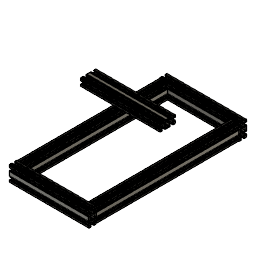
Frame (Autodesk Fusion 360 design; units mm, degrees)
part number: 2026-06-05-11-46-41-486
Autodesk Fusion 360 part; units mm, degrees
(part 1 of 2)
ref_plane "WorkPlane1" through (0, 20, 0) normal (0, 1, 0) x (0, 0, 1)
sketch "Sketch4" plane through (0, 20, 0) normal (0, 1, 0) x (1, 0, 0)
  line L0 (5.5, -26.5607) -> (5.5, -29.7925)
  line L1 (18.5, -27) -> (18.5, -24.05)
  line L2 (6.5607, -34.5) -> (9.7925, -34.5)
  line L3 (0, -26.5) -> (0, -13.5)
  line L4 (0.5, -27) -> (0.5, -26.5)
  line L5 (15.95, -17.0107) -> (15.95, -22.9893)
  line L6 (0, -33.5) -> (0.5, -33.5)
  line L7 (13.4393, -34.5) -> (10.2075, -34.5)
  line L8 (20, -33.5) -> (19.5, -33.5)
  line L9 (13.5, -40) -> (13.5, -39.5)
  line L10 (18.5, -35.95) -> (17.0107, -35.95)
  line L11 (2.9893, -35.95) -> (5.5, -33.4393)
  line L12 (0, -38.5) -> (0, -33.5)
  line L13 (19.5, -33) -> (18.5, -33)
  line L14 (4.05, -38.5) -> (4.05, -37.0107)
  line L15 (15.95, -22.9893) -> (13.4393, -25.5)
  line L16 (4.05, -17.0107) -> (4.05, -22.9893)
  line L17 (1.5, -24.05) -> (2.9893, -24.05)
  line L18 (15.95, -38.5) -> (15.95, -37.0107)
  line L19 (7, -38.5) -> (4.05, -38.5)
  line L20 (19.5, -26.5) -> (19.5, -27)
  line L21 (19.5, -33) -> (19.5, -33.5)
  line L22 (18.5, -33) -> (18.5, -35.95)
  line L23 (13, -39.5) -> (13, -38.5)
  line L24 (6.5, -40) -> (1.5, -40)
  line L25 (20, -33.5) -> (20, -38.5)
  line L26 (14.5, -33.4393) -> (14.5, -30.2075)
  line L27 (15.95, -37.0107) -> (13.4393, -34.5)
  line L28 (18.5, -24.05) -> (17.0107, -24.05)
  line L29 (5.5, -33.4393) -> (5.5, -30.2075)
  line L30 (7, -39.5) -> (6.5, -39.5)
  line L31 (4.05, -22.9893) -> (6.5607, -25.5)
  line L32 (17.0107, -35.95) -> (14.5, -33.4393)
  line L33 (0, -26.5) -> (0.5, -26.5)
  line L34 (1.5, -33) -> (1.5, -35.95)
  line L35 (1.5, -35.95) -> (2.9893, -35.95)
  line L36 (13, -38.5) -> (15.95, -38.5)
  line L37 (0.5, -33.5) -> (0.5, -33)
  line L38 (6.5607, -25.5) -> (9.7925, -25.5)
  line L39 (13.5, -39.5) -> (13, -39.5)
  line L40 (2.9893, -24.05) -> (5.5, -26.5607)
  line L41 (20, -26.5) -> (19.5, -26.5)
  line L42 (7, -39.5) -> (7, -38.5)
  line L43 (6.5, -40) -> (6.5, -39.5)
  line L44 (1.5, -27) -> (1.5, -24.05)
  line L45 (4.05, -37.0107) -> (6.5607, -34.5)
  line L46 (19.5, -27) -> (18.5, -27)
  line L47 (0.5, -33) -> (1.5, -33)
  line L48 (20, -13.5) -> (20, -26.5)
  line L49 (17.0107, -24.05) -> (14.5, -26.5607)
  line L50 (0.5, -27) -> (1.5, -27)
  line L51 (18.5, -40) -> (13.5, -40)
  line L52 (13.4393, -25.5) -> (10.2075, -25.5)
  line L53 (14.5, -26.5607) -> (14.5, -29.7925)
  line L54 (6.5, 0) -> (6.5, -0.5)
  line L55 (13, -0.5) -> (13.5, -0.5)
  line L56 (0.5, -7) -> (0.5, -6.5)
  line L57 (6.5607, -14.5) -> (9.7925, -14.5)
  line L58 (5.5, -13.4393) -> (5.5, -10.2075)
  line L59 (14.5, -13.4393) -> (14.5, -10.2075)
  line L60 (13.4393, -5.5) -> (10.2075, -5.5)
  line L61 (20, -1.5) -> (20, -6.5)
  line L62 (0, -6.5) -> (0.5, -6.5)
  line L63 (15.95, -17.0107) -> (13.4393, -14.5)
  line L64 (1.5, -7) -> (1.5, -4.05)
  line L65 (13.5, 0) -> (13.5, -0.5)
  line L66 (6.5607, -5.5) -> (9.7925, -5.5)
  line L67 (18.5, -4.05) -> (17.0107, -4.05)
  line L68 (7, -0.5) -> (7, -1.5)
  line L69 (4.05, -2.9893) -> (6.5607, -5.5)
  line L70 (6.5, -0.5) -> (7, -0.5)
  line L71 (19.5, -6.5) -> (19.5, -7)
  line L72 (13, -1.5) -> (15.95, -1.5)
  line L73 (0.5, -7) -> (1.5, -7)
  line L74 (19.5, -7) -> (18.5, -7)
  line L75 (13.5, 0) -> (18.5, 0)
  line L76 (14.5, -6.5607) -> (14.5, -9.7925)
  line L77 (18.5, -13) -> (18.5, -15.95)
  line L78 (19.5, -13) -> (18.5, -13)
  line L79 (1.5, 0) -> (6.5, 0)
  line L80 (18.5, -15.95) -> (17.0107, -15.95)
  line L81 (1.5, -15.95) -> (2.9893, -15.95)
  line L82 (19.5, -13) -> (19.5, -13.5)
  line L83 (15.95, -2.9893) -> (13.4393, -5.5)
  line L84 (0.5, -13) -> (1.5, -13)
  line L85 (1.5, -4.05) -> (2.9893, -4.05)
  line L86 (18.5, -7) -> (18.5, -4.05)
  line L87 (1.5, -13) -> (1.5, -15.95)
  line L88 (4.05, -17.0107) -> (6.5607, -14.5)
  line L89 (2.9893, -15.95) -> (5.5, -13.4393)
  line L90 (13.4393, -14.5) -> (10.2075, -14.5)
  line L91 (7, -1.5) -> (4.05, -1.5)
  line L92 (13, -0.5) -> (13, -1.5)
  line L93 (17.0107, -4.05) -> (14.5, -6.5607)
  line L94 (15.95, -1.5) -> (15.95, -2.9893)
  line L95 (20, -6.5) -> (19.5, -6.5)
  line L96 (17.0107, -15.95) -> (14.5, -13.4393)
  line L97 (0.5, -13.5) -> (0.5, -13)
  line L98 (20, -13.5) -> (19.5, -13.5)
  line L99 (2.9893, -4.05) -> (5.5, -6.5607)
  line L100 (0, -6.5) -> (0, -1.5)
  line L101 (0, -13.5) -> (0.5, -13.5)
  line L102 (5.5, -6.5607) -> (5.5, -9.7925)
  line L103 (4.05, -1.5) -> (4.05, -2.9893)
  circle A0 centre (10, -30) radius 2.74
  circle A1 centre (10, -10) radius 2.74
  arc A2 (9.7925, -25.5) -> (10.2075, -25.5) centre (10, -25.5) ccw
  arc A3 (18.5, -40) -> (20, -38.5) centre (18.5, -38.5) ccw
  arc A4 (14.5, -29.7925) -> (14.5, -30.2075) centre (14.5, -30) ccw
  arc A5 (0, -38.5) -> (1.5, -40) centre (1.5, -38.5) ccw
  arc A6 (5.5, -30.2075) -> (5.5, -29.7925) centre (5.5, -30) ccw
  arc A7 (10.2075, -34.5) -> (9.7925, -34.5) centre (10, -34.5) ccw
  arc A8 (9.7925, -5.5) -> (10.2075, -5.5) centre (10, -5.5) ccw
  arc A9 (20, -1.5) -> (18.5, 0) centre (18.5, -1.5) ccw
  arc A10 (10.2075, -14.5) -> (9.7925, -14.5) centre (10, -14.5) ccw
  arc A11 (5.5, -10.2075) -> (5.5, -9.7925) centre (5.5, -10) ccw
  arc A12 (14.5, -9.7925) -> (14.5, -10.2075) centre (14.5, -10) ccw
  arc A13 (1.5, 0) -> (0, -1.5) centre (1.5, -1.5) ccw
  line L104 (184.05, -17.0107) -> (184.05, -22.9893)
  line L105 (200, -13.5) -> (200, -26.5)
  line L106 (180, -26.5) -> (180, -13.5)
  line L107 (180.5, -7) -> (180.5, -6.5)
  line L108 (186.5, -40) -> (186.5, -39.5)
  line L109 (200, -26.5) -> (199.5, -26.5)
  line L110 (180.5, -33) -> (181.5, -33)
  line L111 (180, -6.5) -> (180, -1.5)
  line L112 (193.4393, -34.5) -> (190.2075, -34.5)
  line L113 (185.5, -13.4393) -> (185.5, -10.2075)
  line L114 (193, -1.5) -> (195.95, -1.5)
  line L115 (182.9893, -35.95) -> (185.5, -33.4393)
  arc A14 (190.2075, -34.5) -> (189.7925, -34.5) centre (190, -34.5) ccw
  line L116 (181.5, -35.95) -> (182.9893, -35.95)
  line L117 (180, -13.5) -> (180.5, -13.5)
  line L118 (181.5, -15.95) -> (182.9893, -15.95)
  line L119 (186.5, -0.5) -> (187, -0.5)
  line L120 (193.5, -39.5) -> (193, -39.5)
  arc A15 (194.5, -9.7925) -> (194.5, -10.2075) centre (194.5, -10) ccw
  line L121 (199.5, -33) -> (199.5, -33.5)
  line L122 (198.5, -13) -> (198.5, -15.95)
  line L123 (195.95, -17.0107) -> (193.4393, -14.5)
  line L124 (197.0107, -24.05) -> (194.5, -26.5607)
  line L125 (180.5, -13) -> (181.5, -13)
  line L126 (199.5, -7) -> (198.5, -7)
  line L127 (181.5, 0) -> (186.5, 0)
  line L128 (180.5, -27) -> (181.5, -27)
  line L129 (181.5, -27) -> (181.5, -24.05)
  line L130 (185.5, -26.5607) -> (185.5, -29.7925)
  line L131 (197.0107, -15.95) -> (194.5, -13.4393)
  line L132 (199.5, -26.5) -> (199.5, -27)
  line L133 (181.5, -7) -> (181.5, -4.05)
  circle A16 centre (190, -10) radius 2.74
  arc A17 (200, -1.5) -> (198.5, 0) centre (198.5, -1.5) ccw
  arc A18 (198.5, -40) -> (200, -38.5) centre (198.5, -38.5) ccw
  line L134 (195.95, -1.5) -> (195.95, -2.9893)
  line L135 (182.9893, -15.95) -> (185.5, -13.4393)
  line L136 (200, -33.5) -> (200, -38.5)
  line L137 (184.05, -2.9893) -> (186.5607, -5.5)
  line L138 (193.5, -40) -> (193.5, -39.5)
  line L139 (182.9893, -24.05) -> (185.5, -26.5607)
  line L140 (187, -0.5) -> (187, -1.5)
  line L141 (180.5, -13.5) -> (180.5, -13)
  line L142 (186.5, 0) -> (186.5, -0.5)
  arc A19 (185.5, -30.2075) -> (185.5, -29.7925) centre (185.5, -30) ccw
  line L143 (197.0107, -35.95) -> (194.5, -33.4393)
  line L144 (198.5, -24.05) -> (197.0107, -24.05)
  arc A20 (189.7925, -5.5) -> (190.2075, -5.5) centre (190, -5.5) ccw
  line L145 (198.5, -15.95) -> (197.0107, -15.95)
  line L146 (186.5607, -5.5) -> (189.7925, -5.5)
  line L147 (198.5, -7) -> (198.5, -4.05)
  line L148 (198.5, -4.05) -> (197.0107, -4.05)
  line L149 (193, -39.5) -> (193, -38.5)
  arc A21 (185.5, -10.2075) -> (185.5, -9.7925) centre (185.5, -10) ccw
  line L150 (194.5, -13.4393) -> (194.5, -10.2075)
  line L151 (180, -38.5) -> (180, -33.5)
  line L152 (199.5, -33) -> (198.5, -33)
  line L153 (199.5, -13) -> (199.5, -13.5)
  line L154 (184.05, -37.0107) -> (186.5607, -34.5)
  line L155 (180, -26.5) -> (180.5, -26.5)
  line L156 (180, -33.5) -> (180.5, -33.5)
  line L157 (198.5, -35.95) -> (197.0107, -35.95)
  line L158 (193.4393, -5.5) -> (190.2075, -5.5)
  line L159 (180.5, -33.5) -> (180.5, -33)
  line L160 (198.5, -27) -> (198.5, -24.05)
  line L161 (186.5607, -25.5) -> (189.7925, -25.5)
  line L162 (181.5, -4.05) -> (182.9893, -4.05)
  line L163 (199.5, -27) -> (198.5, -27)
  line L164 (180, -6.5) -> (180.5, -6.5)
  line L165 (184.05, -17.0107) -> (186.5607, -14.5)
  line L166 (193, -0.5) -> (193.5, -0.5)
  line L167 (186.5, -40) -> (181.5, -40)
  line L168 (187, -1.5) -> (184.05, -1.5)
  line L169 (194.5, -26.5607) -> (194.5, -29.7925)
  line L170 (199.5, -13) -> (198.5, -13)
  line L171 (181.5, -24.05) -> (182.9893, -24.05)
  line L172 (193.5, 0) -> (198.5, 0)
  line L173 (182.9893, -4.05) -> (185.5, -6.5607)
  line L174 (195.95, -22.9893) -> (193.4393, -25.5)
  line L175 (180.5, -27) -> (180.5, -26.5)
  line L176 (181.5, -13) -> (181.5, -15.95)
  arc A22 (180, -38.5) -> (181.5, -40) centre (181.5, -38.5) ccw
  line L177 (195.95, -2.9893) -> (193.4393, -5.5)
  line L178 (195.95, -38.5) -> (195.95, -37.0107)
  arc A23 (194.5, -29.7925) -> (194.5, -30.2075) centre (194.5, -30) ccw
  line L179 (194.5, -6.5607) -> (194.5, -9.7925)
  line L180 (197.0107, -4.05) -> (194.5, -6.5607)
  line L181 (193.4393, -25.5) -> (190.2075, -25.5)
  line L182 (181.5, -33) -> (181.5, -35.95)
  line L183 (187, -39.5) -> (187, -38.5)
  line L184 (184.05, -22.9893) -> (186.5607, -25.5)
  line L185 (193.4393, -14.5) -> (190.2075, -14.5)
  line L186 (184.05, -1.5) -> (184.05, -2.9893)
  line L187 (200, -13.5) -> (199.5, -13.5)
  line L188 (187, -38.5) -> (184.05, -38.5)
  line L189 (184.05, -38.5) -> (184.05, -37.0107)
  arc A24 (189.7925, -25.5) -> (190.2075, -25.5) centre (190, -25.5) ccw
  line L190 (195.95, -17.0107) -> (195.95, -22.9893)
  line L191 (198.5, -40) -> (193.5, -40)
  line L192 (186.5607, -14.5) -> (189.7925, -14.5)
  line L193 (194.5, -33.4393) -> (194.5, -30.2075)
  circle A25 centre (190, -30) radius 2.74
  line L194 (185.5, -33.4393) -> (185.5, -30.2075)
  line L195 (193, -0.5) -> (193, -1.5)
  line L196 (185.5, -6.5607) -> (185.5, -9.7925)
  arc A26 (181.5, 0) -> (180, -1.5) centre (181.5, -1.5) ccw
  line L197 (198.5, -33) -> (198.5, -35.95)
  line L198 (193, -38.5) -> (195.95, -38.5)
  line L199 (199.5, -6.5) -> (199.5, -7)
  line L200 (187, -39.5) -> (186.5, -39.5)
  line L201 (180.5, -7) -> (181.5, -7)
  line L202 (193.5, 0) -> (193.5, -0.5)
  arc A27 (190.2075, -14.5) -> (189.7925, -14.5) centre (190, -14.5) ccw
  line L203 (195.95, -37.0107) -> (193.4393, -34.5)
  line L204 (200, -33.5) -> (199.5, -33.5)
  line L205 (200, -1.5) -> (200, -6.5)
  line L206 (186.5607, -34.5) -> (189.7925, -34.5)
  line L207 (200, -6.5) -> (199.5, -6.5)
sketch "Sketch5" plane through (0, 0, 0) normal (1, 0, 0) x (0, 1, 0)
  line L0 (5.5, 13.4393) -> (5.5, 10.2075)
  line L1 (18.5, 13) -> (18.5, 15.95)
  line L2 (6.5607, 5.5) -> (9.7925, 5.5)
  line L3 (0, 13.5) -> (0, 26.5)
  line L4 (0.5, 13) -> (0.5, 13.5)
  line L5 (15.95, 22.9893) -> (15.95, 17.0107)
  line L6 (0, 6.5) -> (0.5, 6.5)
  line L7 (13.4393, 5.5) -> (10.2075, 5.5)
  line L8 (20, 6.5) -> (19.5, 6.5)
  line L9 (13.5, 0) -> (13.5, 0.5)
  line L10 (18.5, 4.05) -> (17.0107, 4.05)
  line L11 (2.9893, 4.05) -> (5.5, 6.5607)
  line L12 (0, 1.5) -> (0, 6.5)
  line L13 (19.5, 7) -> (18.5, 7)
  line L14 (4.05, 1.5) -> (4.05, 2.9893)
  line L15 (15.95, 17.0107) -> (13.4393, 14.5)
  line L16 (4.05, 22.9893) -> (4.05, 17.0107)
  line L17 (1.5, 15.95) -> (2.9893, 15.95)
  line L18 (15.95, 1.5) -> (15.95, 2.9893)
  line L19 (7, 1.5) -> (4.05, 1.5)
  line L20 (19.5, 13.5) -> (19.5, 13)
  line L21 (19.5, 7) -> (19.5, 6.5)
  line L22 (18.5, 7) -> (18.5, 4.05)
  line L23 (13, 0.5) -> (13, 1.5)
  line L24 (6.5, 0) -> (1.5, 0)
  line L25 (20, 6.5) -> (20, 1.5)
  line L26 (14.5, 6.5607) -> (14.5, 9.7925)
  line L27 (15.95, 2.9893) -> (13.4393, 5.5)
  line L28 (18.5, 15.95) -> (17.0107, 15.95)
  line L29 (5.5, 6.5607) -> (5.5, 9.7925)
  line L30 (7, 0.5) -> (6.5, 0.5)
  line L31 (4.05, 17.0107) -> (6.5607, 14.5)
  line L32 (17.0107, 4.05) -> (14.5, 6.5607)
  line L33 (0, 13.5) -> (0.5, 13.5)
  line L34 (1.5, 7) -> (1.5, 4.05)
  line L35 (1.5, 4.05) -> (2.9893, 4.05)
  line L36 (13, 1.5) -> (15.95, 1.5)
  line L37 (0.5, 6.5) -> (0.5, 7)
  line L38 (6.5607, 14.5) -> (9.7925, 14.5)
  line L39 (13.5, 0.5) -> (13, 0.5)
  line L40 (2.9893, 15.95) -> (5.5, 13.4393)
  line L41 (20, 13.5) -> (19.5, 13.5)
  line L42 (7, 0.5) -> (7, 1.5)
  line L43 (6.5, 0) -> (6.5, 0.5)
  line L44 (1.5, 13) -> (1.5, 15.95)
  line L45 (4.05, 2.9893) -> (6.5607, 5.5)
  line L46 (19.5, 13) -> (18.5, 13)
  line L47 (0.5, 7) -> (1.5, 7)
  line L48 (20, 26.5) -> (20, 13.5)
  line L49 (17.0107, 15.95) -> (14.5, 13.4393)
  line L50 (0.5, 13) -> (1.5, 13)
  line L51 (18.5, 0) -> (13.5, 0)
  line L52 (13.4393, 14.5) -> (10.2075, 14.5)
  line L53 (14.5, 13.4393) -> (14.5, 10.2075)
  line L54 (6.5, 40) -> (6.5, 39.5)
  line L55 (13, 39.5) -> (13.5, 39.5)
  line L56 (0.5, 33) -> (0.5, 33.5)
  line L57 (6.5607, 25.5) -> (9.7925, 25.5)
  line L58 (5.5, 26.5607) -> (5.5, 29.7925)
  line L59 (14.5, 26.5607) -> (14.5, 29.7925)
  line L60 (13.4393, 34.5) -> (10.2075, 34.5)
  line L61 (20, 38.5) -> (20, 33.5)
  line L62 (0, 33.5) -> (0.5, 33.5)
  line L63 (15.95, 22.9893) -> (13.4393, 25.5)
  line L64 (1.5, 33) -> (1.5, 35.95)
  line L65 (13.5, 40) -> (13.5, 39.5)
  line L66 (6.5607, 34.5) -> (9.7925, 34.5)
  line L67 (18.5, 35.95) -> (17.0107, 35.95)
  line L68 (7, 39.5) -> (7, 38.5)
  line L69 (4.05, 37.0107) -> (6.5607, 34.5)
  line L70 (6.5, 39.5) -> (7, 39.5)
  line L71 (19.5, 33.5) -> (19.5, 33)
  line L72 (13, 38.5) -> (15.95, 38.5)
  line L73 (0.5, 33) -> (1.5, 33)
  line L74 (19.5, 33) -> (18.5, 33)
  line L75 (13.5, 40) -> (18.5, 40)
  line L76 (14.5, 33.4393) -> (14.5, 30.2075)
  line L77 (18.5, 27) -> (18.5, 24.05)
  line L78 (19.5, 27) -> (18.5, 27)
  line L79 (1.5, 40) -> (6.5, 40)
  line L80 (18.5, 24.05) -> (17.0107, 24.05)
  line L81 (1.5, 24.05) -> (2.9893, 24.05)
  line L82 (19.5, 27) -> (19.5, 26.5)
  line L83 (15.95, 37.0107) -> (13.4393, 34.5)
  line L84 (0.5, 27) -> (1.5, 27)
  line L85 (1.5, 35.95) -> (2.9893, 35.95)
  line L86 (18.5, 33) -> (18.5, 35.95)
  line L87 (1.5, 27) -> (1.5, 24.05)
  line L88 (4.05, 22.9893) -> (6.5607, 25.5)
  line L89 (2.9893, 24.05) -> (5.5, 26.5607)
  line L90 (13.4393, 25.5) -> (10.2075, 25.5)
  line L91 (7, 38.5) -> (4.05, 38.5)
  line L92 (13, 39.5) -> (13, 38.5)
  line L93 (17.0107, 35.95) -> (14.5, 33.4393)
  line L94 (15.95, 38.5) -> (15.95, 37.0107)
  line L95 (20, 33.5) -> (19.5, 33.5)
  line L96 (17.0107, 24.05) -> (14.5, 26.5607)
  line L97 (0.5, 26.5) -> (0.5, 27)
  line L98 (20, 26.5) -> (19.5, 26.5)
  line L99 (2.9893, 35.95) -> (5.5, 33.4393)
  line L100 (0, 33.5) -> (0, 38.5)
  line L101 (0, 26.5) -> (0.5, 26.5)
  line L102 (5.5, 33.4393) -> (5.5, 30.2075)
  line L103 (4.05, 38.5) -> (4.05, 37.0107)
  circle A0 centre (10, 10) radius 2.74
  circle A1 centre (10, 30) radius 2.74
  arc A2 (9.7925, 14.5) -> (10.2075, 14.5) centre (10, 14.5) ccw
  arc A3 (18.5, 0) -> (20, 1.5) centre (18.5, 1.5) ccw
  arc A4 (14.5, 10.2075) -> (14.5, 9.7925) centre (14.5, 10) ccw
  arc A5 (0, 1.5) -> (1.5, 0) centre (1.5, 1.5) ccw
  arc A6 (5.5, 9.7925) -> (5.5, 10.2075) centre (5.5, 10) ccw
  arc A7 (10.2075, 5.5) -> (9.7925, 5.5) centre (10, 5.5) ccw
  arc A8 (9.7925, 34.5) -> (10.2075, 34.5) centre (10, 34.5) ccw
  arc A9 (20, 38.5) -> (18.5, 40) centre (18.5, 38.5) ccw
  arc A10 (10.2075, 25.5) -> (9.7925, 25.5) centre (10, 25.5) ccw
  arc A11 (5.5, 29.7925) -> (5.5, 30.2075) centre (5.5, 30) ccw
  arc A12 (14.5, 30.2075) -> (14.5, 29.7925) centre (14.5, 30) ccw
  arc A13 (1.5, 40) -> (0, 38.5) centre (1.5, 38.5) ccw
  line L104 (398.5, 35.95) -> (397.0107, 35.95)
  line L105 (398.5, 0) -> (393.5, 0)
  line L106 (393.5, 0.5) -> (393, 0.5)
  arc A14 (389.7925, 34.5) -> (390.2075, 34.5) centre (390, 34.5) ccw
  line L107 (397.0107, 15.95) -> (394.5, 13.4393)
  line L108 (381.5, 13) -> (381.5, 15.95)
  line L109 (393, 0.5) -> (393, 1.5)
  arc A15 (390.2075, 25.5) -> (389.7925, 25.5) centre (390, 25.5) ccw
  line L110 (394.5, 13.4393) -> (394.5, 10.2075)
  line L111 (393.5, 40) -> (398.5, 40)
  line L112 (400, 26.5) -> (400, 13.5)
  line L113 (399.5, 7) -> (398.5, 7)
  line L114 (398.5, 4.05) -> (397.0107, 4.05)
  line L115 (398.5, 15.95) -> (397.0107, 15.95)
  line L116 (399.5, 27) -> (399.5, 26.5)
  line L117 (382.9893, 35.95) -> (385.5, 33.4393)
  line L118 (398.5, 7) -> (398.5, 4.05)
  line L119 (381.5, 40) -> (386.5, 40)
  line L120 (398.5, 24.05) -> (397.0107, 24.05)
  line L121 (382.9893, 15.95) -> (385.5, 13.4393)
  arc A16 (398.5, 0) -> (400, 1.5) centre (398.5, 1.5) ccw
  line L122 (398.5, 27) -> (398.5, 24.05)
  line L123 (400, 26.5) -> (399.5, 26.5)
  line L124 (399.5, 27) -> (398.5, 27)
  arc A17 (381.5, 40) -> (380, 38.5) centre (381.5, 38.5) ccw
  line L125 (384.05, 2.9893) -> (386.5607, 5.5)
  line L126 (395.95, 1.5) -> (395.95, 2.9893)
  line L127 (380, 13.5) -> (380.5, 13.5)
  line L128 (393, 38.5) -> (395.95, 38.5)
  line L129 (393.4393, 5.5) -> (390.2075, 5.5)
  line L130 (380.5, 26.5) -> (380.5, 27)
  line L131 (380, 33.5) -> (380.5, 33.5)
  arc A18 (385.5, 9.7925) -> (385.5, 10.2075) centre (385.5, 10) ccw
  arc A19 (390.2075, 5.5) -> (389.7925, 5.5) centre (390, 5.5) ccw
  arc A20 (394.5, 30.2075) -> (394.5, 29.7925) centre (394.5, 30) ccw
  line L132 (393.4393, 25.5) -> (390.2075, 25.5)
  line L133 (386.5, 40) -> (386.5, 39.5)
  line L134 (385.5, 26.5607) -> (385.5, 29.7925)
  line L135 (395.95, 38.5) -> (395.95, 37.0107)
  line L136 (382.9893, 4.05) -> (385.5, 6.5607)
  line L137 (400, 33.5) -> (399.5, 33.5)
  line L138 (399.5, 7) -> (399.5, 6.5)
  line L139 (382.9893, 24.05) -> (385.5, 26.5607)
  line L140 (400, 13.5) -> (399.5, 13.5)
  line L141 (399.5, 13.5) -> (399.5, 13)
  line L142 (380, 1.5) -> (380, 6.5)
  line L143 (400, 6.5) -> (399.5, 6.5)
  line L144 (386.5, 0) -> (381.5, 0)
  line L145 (398.5, 13) -> (398.5, 15.95)
  line L146 (395.95, 2.9893) -> (393.4393, 5.5)
  line L147 (387, 38.5) -> (384.05, 38.5)
  line L148 (393.4393, 34.5) -> (390.2075, 34.5)
  line L149 (386.5607, 25.5) -> (389.7925, 25.5)
  line L150 (386.5607, 14.5) -> (389.7925, 14.5)
  line L151 (387, 0.5) -> (387, 1.5)
  line L152 (384.05, 1.5) -> (384.05, 2.9893)
  line L153 (385.5, 6.5607) -> (385.5, 9.7925)
  line L154 (385.5, 13.4393) -> (385.5, 10.2075)
  circle A21 centre (390, 30) radius 2.74
  line L155 (387, 39.5) -> (387, 38.5)
  line L156 (397.0107, 4.05) -> (394.5, 6.5607)
  line L157 (393, 39.5) -> (393.5, 39.5)
  line L158 (397.0107, 35.95) -> (394.5, 33.4393)
  arc A22 (385.5, 29.7925) -> (385.5, 30.2075) centre (385.5, 30) ccw
  arc A23 (394.5, 10.2075) -> (394.5, 9.7925) centre (394.5, 10) ccw
  line L159 (384.05, 22.9893) -> (386.5607, 25.5)
  line L160 (395.95, 22.9893) -> (393.4393, 25.5)
  line L161 (394.5, 26.5607) -> (394.5, 29.7925)
  line L162 (393.5, 0) -> (393.5, 0.5)
  line L163 (380, 26.5) -> (380.5, 26.5)
  line L164 (384.05, 17.0107) -> (386.5607, 14.5)
  line L165 (380.5, 13) -> (381.5, 13)
  line L166 (385.5, 33.4393) -> (385.5, 30.2075)
  line L167 (400, 38.5) -> (400, 33.5)
  line L168 (386.5, 39.5) -> (387, 39.5)
  arc A24 (389.7925, 14.5) -> (390.2075, 14.5) centre (390, 14.5) ccw
  line L169 (381.5, 35.95) -> (382.9893, 35.95)
  line L170 (397.0107, 24.05) -> (394.5, 26.5607)
  line L171 (393, 1.5) -> (395.95, 1.5)
  line L172 (386.5607, 34.5) -> (389.7925, 34.5)
  line L173 (395.95, 37.0107) -> (393.4393, 34.5)
  circle A25 centre (390, 10) radius 2.74
  line L174 (399.5, 33) -> (398.5, 33)
  line L175 (395.95, 22.9893) -> (395.95, 17.0107)
  line L176 (380.5, 33) -> (381.5, 33)
  line L177 (393.4393, 14.5) -> (390.2075, 14.5)
  line L178 (381.5, 4.05) -> (382.9893, 4.05)
  line L179 (380.5, 7) -> (381.5, 7)
  line L180 (384.05, 38.5) -> (384.05, 37.0107)
  line L181 (380.5, 27) -> (381.5, 27)
  line L182 (386.5607, 5.5) -> (389.7925, 5.5)
  line L183 (381.5, 24.05) -> (382.9893, 24.05)
  line L184 (381.5, 27) -> (381.5, 24.05)
  arc A26 (380, 1.5) -> (381.5, 0) centre (381.5, 1.5) ccw
  line L185 (394.5, 33.4393) -> (394.5, 30.2075)
  line L186 (393.5, 40) -> (393.5, 39.5)
  line L187 (380, 13.5) -> (380, 26.5)
  line L188 (380, 6.5) -> (380.5, 6.5)
  line L189 (380, 33.5) -> (380, 38.5)
  line L190 (387, 0.5) -> (386.5, 0.5)
  line L191 (381.5, 7) -> (381.5, 4.05)
  line L192 (380.5, 33) -> (380.5, 33.5)
  line L193 (381.5, 15.95) -> (382.9893, 15.95)
  line L194 (394.5, 6.5607) -> (394.5, 9.7925)
  line L195 (393, 39.5) -> (393, 38.5)
  line L196 (386.5, 0) -> (386.5, 0.5)
  line L197 (395.95, 17.0107) -> (393.4393, 14.5)
  line L198 (381.5, 33) -> (381.5, 35.95)
  line L199 (384.05, 37.0107) -> (386.5607, 34.5)
  line L200 (400, 6.5) -> (400, 1.5)
  line L201 (398.5, 33) -> (398.5, 35.95)
  line L202 (380.5, 13) -> (380.5, 13.5)
  line L203 (387, 1.5) -> (384.05, 1.5)
  line L204 (399.5, 33.5) -> (399.5, 33)
  line L205 (380.5, 6.5) -> (380.5, 7)
  line L206 (384.05, 22.9893) -> (384.05, 17.0107)
  line L207 (399.5, 13) -> (398.5, 13)
  arc A27 (400, 38.5) -> (398.5, 40) centre (398.5, 38.5) ccw
ref_plane "WorkPlane2" through (0, 0, 40) normal (0, 0, 1) x (1, 0, 0)
sketch "Sketch6" plane through (0, 0, 40) normal (0, 0, 1) x (1, 0, 0)
  line L0 (5.5, 193.4393) -> (5.5, 190.2075)
  line L1 (18.5, 193) -> (18.5, 195.95)
  line L2 (6.5607, 185.5) -> (9.7925, 185.5)
  line L3 (0, 193.5) -> (0, 206.5)
  line L4 (0.5, 193) -> (0.5, 193.5)
  line L5 (15.95, 202.9893) -> (15.95, 197.0107)
  line L6 (0, 186.5) -> (0.5, 186.5)
  line L7 (13.4393, 185.5) -> (10.2075, 185.5)
  line L8 (20, 186.5) -> (19.5, 186.5)
  line L9 (13.5, 180) -> (13.5, 180.5)
  line L10 (18.5, 184.05) -> (17.0107, 184.05)
  line L11 (2.9893, 184.05) -> (5.5, 186.5607)
  line L12 (0, 181.5) -> (0, 186.5)
  line L13 (19.5, 187) -> (18.5, 187)
  line L14 (4.05, 181.5) -> (4.05, 182.9893)
  line L15 (15.95, 197.0107) -> (13.4393, 194.5)
  line L16 (4.05, 202.9893) -> (4.05, 197.0107)
  line L17 (1.5, 195.95) -> (2.9893, 195.95)
  line L18 (15.95, 181.5) -> (15.95, 182.9893)
  line L19 (7, 181.5) -> (4.05, 181.5)
  line L20 (19.5, 193.5) -> (19.5, 193)
  line L21 (19.5, 187) -> (19.5, 186.5)
  line L22 (18.5, 187) -> (18.5, 184.05)
  line L23 (13, 180.5) -> (13, 181.5)
  line L24 (6.5, 180) -> (1.5, 180)
  line L25 (20, 186.5) -> (20, 181.5)
  line L26 (14.5, 186.5607) -> (14.5, 189.7925)
  line L27 (15.95, 182.9893) -> (13.4393, 185.5)
  line L28 (18.5, 195.95) -> (17.0107, 195.95)
  line L29 (5.5, 186.5607) -> (5.5, 189.7925)
  line L30 (7, 180.5) -> (6.5, 180.5)
  line L31 (4.05, 197.0107) -> (6.5607, 194.5)
  line L32 (17.0107, 184.05) -> (14.5, 186.5607)
  line L33 (0, 193.5) -> (0.5, 193.5)
  line L34 (1.5, 187) -> (1.5, 184.05)
  line L35 (1.5, 184.05) -> (2.9893, 184.05)
  line L36 (13, 181.5) -> (15.95, 181.5)
  line L37 (0.5, 186.5) -> (0.5, 187)
  line L38 (6.5607, 194.5) -> (9.7925, 194.5)
  line L39 (13.5, 180.5) -> (13, 180.5)
  line L40 (2.9893, 195.95) -> (5.5, 193.4393)
  line L41 (20, 193.5) -> (19.5, 193.5)
  line L42 (7, 180.5) -> (7, 181.5)
  line L43 (6.5, 180) -> (6.5, 180.5)
  line L44 (1.5, 193) -> (1.5, 195.95)
  line L45 (4.05, 182.9893) -> (6.5607, 185.5)
  line L46 (19.5, 193) -> (18.5, 193)
  line L47 (0.5, 187) -> (1.5, 187)
  line L48 (20, 206.5) -> (20, 193.5)
  line L49 (17.0107, 195.95) -> (14.5, 193.4393)
  line L50 (0.5, 193) -> (1.5, 193)
  line L51 (18.5, 180) -> (13.5, 180)
  line L52 (13.4393, 194.5) -> (10.2075, 194.5)
  line L53 (14.5, 193.4393) -> (14.5, 190.2075)
  line L54 (6.5, 220) -> (6.5, 219.5)
  line L55 (13, 219.5) -> (13.5, 219.5)
  line L56 (0.5, 213) -> (0.5, 213.5)
  line L57 (6.5607, 205.5) -> (9.7925, 205.5)
  line L58 (5.5, 206.5607) -> (5.5, 209.7925)
  line L59 (14.5, 206.5607) -> (14.5, 209.7925)
  line L60 (13.4393, 214.5) -> (10.2075, 214.5)
  line L61 (20, 218.5) -> (20, 213.5)
  line L62 (0, 213.5) -> (0.5, 213.5)
  line L63 (15.95, 202.9893) -> (13.4393, 205.5)
  line L64 (1.5, 213) -> (1.5, 215.95)
  line L65 (13.5, 220) -> (13.5, 219.5)
  line L66 (6.5607, 214.5) -> (9.7925, 214.5)
  line L67 (18.5, 215.95) -> (17.0107, 215.95)
  line L68 (7, 219.5) -> (7, 218.5)
  line L69 (4.05, 217.0107) -> (6.5607, 214.5)
  line L70 (6.5, 219.5) -> (7, 219.5)
  line L71 (19.5, 213.5) -> (19.5, 213)
  line L72 (13, 218.5) -> (15.95, 218.5)
  line L73 (0.5, 213) -> (1.5, 213)
  line L74 (19.5, 213) -> (18.5, 213)
  line L75 (13.5, 220) -> (18.5, 220)
  line L76 (14.5, 213.4393) -> (14.5, 210.2075)
  line L77 (18.5, 207) -> (18.5, 204.05)
  line L78 (19.5, 207) -> (18.5, 207)
  line L79 (1.5, 220) -> (6.5, 220)
  line L80 (18.5, 204.05) -> (17.0107, 204.05)
  line L81 (1.5, 204.05) -> (2.9893, 204.05)
  line L82 (19.5, 207) -> (19.5, 206.5)
  line L83 (15.95, 217.0107) -> (13.4393, 214.5)
  line L84 (0.5, 207) -> (1.5, 207)
  line L85 (1.5, 215.95) -> (2.9893, 215.95)
  line L86 (18.5, 213) -> (18.5, 215.95)
  line L87 (1.5, 207) -> (1.5, 204.05)
  line L88 (4.05, 202.9893) -> (6.5607, 205.5)
  line L89 (2.9893, 204.05) -> (5.5, 206.5607)
  line L90 (13.4393, 205.5) -> (10.2075, 205.5)
  line L91 (7, 218.5) -> (4.05, 218.5)
  line L92 (13, 219.5) -> (13, 218.5)
  line L93 (17.0107, 215.95) -> (14.5, 213.4393)
  line L94 (15.95, 218.5) -> (15.95, 217.0107)
  line L95 (20, 213.5) -> (19.5, 213.5)
  line L96 (17.0107, 204.05) -> (14.5, 206.5607)
  line L97 (0.5, 206.5) -> (0.5, 207)
  line L98 (20, 206.5) -> (19.5, 206.5)
  line L99 (2.9893, 215.95) -> (5.5, 213.4393)
  line L100 (0, 213.5) -> (0, 218.5)
  line L101 (0, 206.5) -> (0.5, 206.5)
  line L102 (5.5, 213.4393) -> (5.5, 210.2075)
  line L103 (4.05, 218.5) -> (4.05, 217.0107)
  circle A0 centre (10, 190) radius 2.74
  circle A1 centre (10, 210) radius 2.74
  arc A2 (9.7925, 194.5) -> (10.2075, 194.5) centre (10, 194.5) ccw
  arc A3 (18.5, 180) -> (20, 181.5) centre (18.5, 181.5) ccw
  arc A4 (14.5, 190.2075) -> (14.5, 189.7925) centre (14.5, 190) ccw
  arc A5 (0, 181.5) -> (1.5, 180) centre (1.5, 181.5) ccw
  arc A6 (5.5, 189.7925) -> (5.5, 190.2075) centre (5.5, 190) ccw
  arc A7 (10.2075, 185.5) -> (9.7925, 185.5) centre (10, 185.5) ccw
  arc A8 (9.7925, 214.5) -> (10.2075, 214.5) centre (10, 214.5) ccw
  arc A9 (20, 218.5) -> (18.5, 220) centre (18.5, 218.5) ccw
  arc A10 (10.2075, 205.5) -> (9.7925, 205.5) centre (10, 205.5) ccw
  arc A11 (5.5, 209.7925) -> (5.5, 210.2075) centre (5.5, 210) ccw
  arc A12 (14.5, 210.2075) -> (14.5, 209.7925) centre (14.5, 210) ccw
  arc A13 (1.5, 220) -> (0, 218.5) centre (1.5, 218.5) ccw
  line L104 (299.5, 193) -> (298.5, 193)
  line L105 (299.5, 207) -> (298.5, 207)
  arc A14 (294.5, 190.2075) -> (294.5, 189.7925) centre (294.5, 190) ccw
  line L106 (299.5, 193.5) -> (299.5, 193)
  line L107 (299.5, 213.5) -> (299.5, 213)
  line L108 (294.5, 193.4393) -> (294.5, 190.2075)
  line L109 (298.5, 184.05) -> (297.0107, 184.05)
  line L110 (280, 206.5) -> (280.5, 206.5)
  line L111 (300, 218.5) -> (300, 213.5)
  line L112 (293.4393, 205.5) -> (290.2075, 205.5)
  line L113 (297.0107, 204.05) -> (294.5, 206.5607)
  line L114 (280.5, 206.5) -> (280.5, 207)
  line L115 (299.5, 213) -> (298.5, 213)
  line L116 (287, 219.5) -> (287, 218.5)
  line L117 (299.5, 187) -> (299.5, 186.5)
  line L118 (299.5, 187) -> (298.5, 187)
  line L119 (300, 193.5) -> (299.5, 193.5)
  line L120 (285.5, 206.5607) -> (285.5, 209.7925)
  line L121 (280, 213.5) -> (280.5, 213.5)
  arc A15 (280, 181.5) -> (281.5, 180) centre (281.5, 181.5) ccw
  line L122 (299.5, 207) -> (299.5, 206.5)
  line L123 (280, 193.5) -> (280.5, 193.5)
  line L124 (294.5, 186.5607) -> (294.5, 189.7925)
  line L125 (295.95, 181.5) -> (295.95, 182.9893)
  line L126 (298.5, 207) -> (298.5, 204.05)
  arc A16 (289.7925, 214.5) -> (290.2075, 214.5) centre (290, 214.5) ccw
  line L127 (281.5, 215.95) -> (282.9893, 215.95)
  line L128 (284.05, 218.5) -> (284.05, 217.0107)
  line L129 (284.05, 197.0107) -> (286.5607, 194.5)
  line L130 (280, 186.5) -> (280.5, 186.5)
  line L131 (280.5, 187) -> (281.5, 187)
  line L132 (293, 181.5) -> (295.95, 181.5)
  line L133 (281.5, 207) -> (281.5, 204.05)
  line L134 (298.5, 213) -> (298.5, 215.95)
  arc A17 (290.2075, 185.5) -> (289.7925, 185.5) centre (290, 185.5) ccw
  line L135 (293.5, 220) -> (298.5, 220)
  line L136 (297.0107, 184.05) -> (294.5, 186.5607)
  line L137 (298.5, 204.05) -> (297.0107, 204.05)
  line L138 (297.0107, 215.95) -> (294.5, 213.4393)
  line L139 (280.5, 186.5) -> (280.5, 187)
  line L140 (300, 206.5) -> (299.5, 206.5)
  line L141 (287, 180.5) -> (286.5, 180.5)
  line L142 (298.5, 195.95) -> (297.0107, 195.95)
  line L143 (300, 213.5) -> (299.5, 213.5)
  line L144 (280, 193.5) -> (280, 206.5)
  line L145 (294.5, 206.5607) -> (294.5, 209.7925)
  line L146 (298.5, 187) -> (298.5, 184.05)
  arc A18 (289.7925, 194.5) -> (290.2075, 194.5) centre (290, 194.5) ccw
  line L147 (300, 186.5) -> (300, 181.5)
  line L148 (293.5, 220) -> (293.5, 219.5)
  line L149 (293.4393, 194.5) -> (290.2075, 194.5)
  arc A19 (294.5, 210.2075) -> (294.5, 209.7925) centre (294.5, 210) ccw
  line L150 (287, 218.5) -> (284.05, 218.5)
  line L151 (284.05, 202.9893) -> (286.5607, 205.5)
  line L152 (280, 213.5) -> (280, 218.5)
  line L153 (286.5, 220) -> (286.5, 219.5)
  arc A20 (290.2075, 205.5) -> (289.7925, 205.5) centre (290, 205.5) ccw
  line L154 (280, 181.5) -> (280, 186.5)
  arc A21 (281.5, 220) -> (280, 218.5) centre (281.5, 218.5) ccw
  line L155 (297.0107, 195.95) -> (294.5, 193.4393)
  line L156 (295.95, 218.5) -> (295.95, 217.0107)
  line L157 (286.5607, 185.5) -> (289.7925, 185.5)
  line L158 (293, 180.5) -> (293, 181.5)
  line L159 (293.5, 180) -> (293.5, 180.5)
  line L160 (295.95, 202.9893) -> (295.95, 197.0107)
  line L161 (300, 206.5) -> (300, 193.5)
  line L162 (286.5, 219.5) -> (287, 219.5)
  line L163 (280.5, 213) -> (281.5, 213)
  line L164 (293.5, 180.5) -> (293, 180.5)
  line L165 (293.4393, 185.5) -> (290.2075, 185.5)
  line L166 (281.5, 204.05) -> (282.9893, 204.05)
  line L167 (298.5, 180) -> (293.5, 180)
  line L168 (285.5, 213.4393) -> (285.5, 210.2075)
  line L169 (282.9893, 184.05) -> (285.5, 186.5607)
  line L170 (293, 218.5) -> (295.95, 218.5)
  line L171 (293.4393, 214.5) -> (290.2075, 214.5)
  line L172 (298.5, 193) -> (298.5, 195.95)
  line L173 (293, 219.5) -> (293, 218.5)
  line L174 (280.5, 213) -> (280.5, 213.5)
  line L175 (280.5, 207) -> (281.5, 207)
  line L176 (284.05, 217.0107) -> (286.5607, 214.5)
  line L177 (293, 219.5) -> (293.5, 219.5)
  arc A22 (298.5, 180) -> (300, 181.5) centre (298.5, 181.5) ccw
  line L178 (284.05, 202.9893) -> (284.05, 197.0107)
  line L179 (280.5, 193) -> (281.5, 193)
  arc A23 (300, 218.5) -> (298.5, 220) centre (298.5, 218.5) ccw
  line L180 (281.5, 220) -> (286.5, 220)
  arc A24 (285.5, 209.7925) -> (285.5, 210.2075) centre (285.5, 210) ccw
  line L181 (284.05, 181.5) -> (284.05, 182.9893)
  line L182 (287, 181.5) -> (284.05, 181.5)
  line L183 (282.9893, 204.05) -> (285.5, 206.5607)
  line L184 (284.05, 182.9893) -> (286.5607, 185.5)
  arc A25 (285.5, 189.7925) -> (285.5, 190.2075) centre (285.5, 190) ccw
  line L185 (298.5, 215.95) -> (297.0107, 215.95)
  line L186 (281.5, 213) -> (281.5, 215.95)
  line L187 (280.5, 193) -> (280.5, 193.5)
  line L188 (282.9893, 195.95) -> (285.5, 193.4393)
  line L189 (285.5, 193.4393) -> (285.5, 190.2075)
  line L190 (285.5, 186.5607) -> (285.5, 189.7925)
  line L191 (287, 180.5) -> (287, 181.5)
  line L192 (281.5, 195.95) -> (282.9893, 195.95)
  line L193 (281.5, 187) -> (281.5, 184.05)
  line L194 (286.5, 180) -> (281.5, 180)
  circle A26 centre (290, 210) radius 2.74
  line L195 (286.5607, 194.5) -> (289.7925, 194.5)
  circle A27 centre (290, 190) radius 2.74
  line L196 (286.5607, 214.5) -> (289.7925, 214.5)
  line L197 (286.5607, 205.5) -> (289.7925, 205.5)
  line L198 (295.95, 202.9893) -> (293.4393, 205.5)
  line L199 (295.95, 197.0107) -> (293.4393, 194.5)
  line L200 (281.5, 193) -> (281.5, 195.95)
  line L201 (295.95, 182.9893) -> (293.4393, 185.5)
  line L202 (282.9893, 215.95) -> (285.5, 213.4393)
  line L203 (281.5, 184.05) -> (282.9893, 184.05)
  line L204 (300, 186.5) -> (299.5, 186.5)
  line L205 (295.95, 217.0107) -> (293.4393, 214.5)
  line L206 (286.5, 180) -> (286.5, 180.5)
  line L207 (294.5, 213.4393) -> (294.5, 210.2075)
extrude "Extrude1" add sketch "Sketch4" along normal blind 360 contours L0 L1 L2 L3 L4 L6 L7 L8 L9 L10 L11 L12 L13 L14 L17 L18 L19 L20 L21 L22 L23 L24 L25 L26 L27 L28 L29 L30 L32 L33 L34 L35 L36 L37 L39 L40 L41 L42 L43 L44 L45 L46 L47 L48 L49 L50 L51 L53 L54 L55 L56 L58 L59 L60 L61 L62 L64 L65 L66 L67 L68 L69 L70 L71 L72 L73 L74 L75 L76 L77 L78 L79 L80 L81 L82 L83 L84 L85 L86 L87 L89 L91 L92 L93 L94 L95 L96 L97 L98 L99 L100 L101 L102 L103 A3 A4 A5 A6 A7 A8 A9 A11 A12 A13 makes body 1
extrude "Extrude2" add sketch "Sketch5" along normal blind 200 separate body contours L0 L1 L2 L3 L4 L6 L7 L8 L9 L10 L11 L12 L13 L14 L17 L18 L19 L20 L21 L22 L23 L24 L25 L26 L27 L28 L29 L30 L32 L33 L34 L35 L36 L37 L39 L40 L41 L42 L43 L44 L45 L46 L47 L48 L49 L50 L51 L53 L54 L55 L56 L58 L59 L60 L61 L62 L64 L65 L66 L67 L68 L69 L70 L71 L72 L73 L74 L75 L76 L77 L78 L79 L80 L81 L82 L83 L84 L85 L86 L87 L89 L91 L92 L93 L94 L95 L96 L97 L98 L99 L100 L101 L102 L103 A3 A4 A5 A6 A7 A8 A9 A11 A12 A13 makes body 2
extrude "Extrude3" add sketch "Sketch5" along normal blind 200 separate body contours L104 L105 L106 A14 L107 L108 L109 L110 L111 L112 L113 L114 L115 L116 L117 L118 L119 L120 L121 A16 L122 L123 L124 A17 L125 L126 L127 L128 L129 L130 L131 A18 A19 A20 L133 L134 L135 L136 L137 L138 L139 L140 L141 L142 L143 L144 L145 L146 L147 L148 L151 L152 L153 L154 L155 L156 L157 L158 A22 A23 L161 L162 L163 L165 L166 L167 L168 L169 L170 L171 L172 L173 L174 L176 L178 L179 L180 L181 L182 L183 L184 A26 L185 L186 L187 L188 L189 L190 L191 L192 L193 L194 L195 L196 L198 L199 L200 L201 L202 L203 L204 L205 L207 A27 makes body 3
extrude "Extrude4" add sketch "Sketch4" along normal blind 360 separate body contours L105 L106 L107 L108 L109 L110 L111 L112 L113 L114 L115 A14 L116 L117 L118 L119 L120 A15 L121 L122 L124 L125 L126 L127 L128 L129 L130 L131 L132 L133 A17 A18 L134 L135 L136 L137 L138 L139 L140 L141 L142 A19 L143 L144 A20 L145 L146 L147 L148 L149 A21 L150 L151 L152 L153 L154 L155 L156 L157 L158 L159 L160 L162 L163 L164 L166 L167 L168 L169 L170 L171 L172 L173 L175 L176 A22 L177 L178 A23 L179 L180 L182 L183 L186 L187 L188 L189 L191 L193 L194 L195 L196 A26 L197 L198 L199 L200 L201 L202 L203 L204 L205 L206 L207 makes body 4
extrude "Extrude5" add sketch "Sketch6" along normal blind 80 separate body contours L0 L1 L2 L3 L4 L6 L7 L8 L9 L10 L11 L12 L13 L14 L17 L18 L19 L20 L21 L22 L23 L24 L25 L26 L27 L28 L29 L30 L32 L33 L34 L35 L36 L37 L39 L40 L41 L42 L43 L44 L45 L46 L47 L48 L49 L50 L51 L53 L54 L55 L56 L58 L59 L60 L61 L62 L64 L65 L66 L67 L68 L69 L70 L71 L72 L73 L74 L75 L76 L77 L78 L79 L80 L81 L82 L83 L84 L85 L86 L87 L89 L91 L92 L93 L94 L95 L96 L97 L98 L99 L100 L101 L102 L103 A3 A4 A5 A6 A7 A8 A9 A11 A12 A13 makes body 5
extrude "Extrude6" add sketch "Sketch6" along normal blind 80 separate body contours L104 L105 A14 L106 L107 L108 L109 L110 L111 L113 L114 L115 L116 L117 L118 L119 L120 L121 A15 L122 L123 L124 L125 L126 A16 L127 L128 L130 L131 L132 L133 L134 A17 L135 L136 L137 L138 L139 L140 L141 L142 L143 L144 L145 L146 L147 L148 A19 L150 L152 L153 L154 A21 L155 L156 L157 L158 L159 L161 L162 L163 L164 L165 L166 L167 L168 L169 L170 L171 L172 L173 L174 L175 L176 L177 A22 L179 A23 L180 A24 L181 L182 L183 L184 A25 L185 L186 L187 L188 L189 L190 L191 L192 L193 L194 L196 L200 L201 L202 L203 L204 L205 L206 L207 makes body 6
sketch "Sketch7" plane through (0, 0, 0) normal (1, 0, 0) x (0, 1, 0)
  line L0 (206.5607, 125.5) -> (209.7925, 125.5)
  line L1 (207, 138.5) -> (204.05, 138.5)
  line L2 (214.5, 126.5607) -> (214.5, 129.7925)
  line L3 (206.5, 120) -> (193.5, 120)
  line L4 (207, 120.5) -> (206.5, 120.5)
  line L5 (213.5, 120) -> (213.5, 120.5)
  line L6 (214.5, 133.4393) -> (214.5, 130.2075)
  line L7 (213.5, 140) -> (213.5, 139.5)
  line L8 (220, 133.5) -> (219.5, 133.5)
  line L9 (215.95, 138.5) -> (215.95, 137.0107)
  line L10 (215.95, 122.9893) -> (213.4393, 125.5)
  line L11 (218.5, 120) -> (213.5, 120)
  line L12 (213, 139.5) -> (213, 138.5)
  line L13 (218.5, 124.05) -> (217.0107, 124.05)
  line L14 (202.9893, 135.95) -> (205.5, 133.4393)
  line L15 (204.05, 121.5) -> (204.05, 122.9893)
  line L16 (218.5, 135.95) -> (217.0107, 135.95)
  line L17 (218.5, 127) -> (218.5, 124.05)
  line L18 (206.5, 139.5) -> (207, 139.5)
  line L19 (213, 139.5) -> (213.5, 139.5)
  line L20 (213, 138.5) -> (215.95, 138.5)
  line L21 (219.5, 133) -> (218.5, 133)
  line L22 (220, 126.5) -> (220, 121.5)
  line L23 (213.5, 140) -> (218.5, 140)
  line L24 (213.4393, 134.5) -> (210.2075, 134.5)
  line L25 (217.0107, 135.95) -> (214.5, 133.4393)
  line L26 (204.05, 138.5) -> (204.05, 137.0107)
  line L27 (213.4393, 125.5) -> (210.2075, 125.5)
  line L28 (219.5, 127) -> (219.5, 126.5)
  line L29 (202.9893, 124.05) -> (205.5, 126.5607)
  line L30 (215.95, 137.0107) -> (213.4393, 134.5)
  line L31 (206.5, 120) -> (206.5, 120.5)
  line L32 (213, 121.5) -> (215.95, 121.5)
  line L33 (215.95, 121.5) -> (215.95, 122.9893)
  line L34 (218.5, 133) -> (218.5, 135.95)
  line L35 (213.5, 120.5) -> (213, 120.5)
  line L36 (205.5, 126.5607) -> (205.5, 129.7925)
  line L37 (219.5, 133.5) -> (219.5, 133)
  line L38 (204.05, 122.9893) -> (206.5607, 125.5)
  line L39 (206.5, 140) -> (206.5, 139.5)
  line L40 (219.5, 127) -> (218.5, 127)
  line L41 (220, 126.5) -> (219.5, 126.5)
  line L42 (207, 121.5) -> (204.05, 121.5)
  line L43 (217.0107, 124.05) -> (214.5, 126.5607)
  line L44 (207, 139.5) -> (207, 138.5)
  line L45 (213, 120.5) -> (213, 121.5)
  line L46 (193.5, 140) -> (206.5, 140)
  line L47 (204.05, 137.0107) -> (206.5607, 134.5)
  line L48 (207, 120.5) -> (207, 121.5)
  line L49 (220, 138.5) -> (220, 133.5)
  line L50 (205.5, 133.4393) -> (205.5, 130.2075)
  line L51 (206.5607, 134.5) -> (209.7925, 134.5)
  line L52 (180, 126.5) -> (180.5, 126.5)
  line L53 (180.5, 133) -> (180.5, 133.5)
  line L54 (187, 120.5) -> (186.5, 120.5)
  line L55 (194.5, 126.5607) -> (194.5, 129.7925)
  line L56 (193.4393, 125.5) -> (190.2075, 125.5)
  line L57 (193.4393, 134.5) -> (190.2075, 134.5)
  line L58 (185.5, 133.4393) -> (185.5, 130.2075)
  line L59 (181.5, 140) -> (186.5, 140)
  line L60 (186.5, 120) -> (186.5, 120.5)
  line L61 (197.0107, 135.95) -> (194.5, 133.4393)
  line L62 (187, 121.5) -> (184.05, 121.5)
  line L63 (180, 133.5) -> (180.5, 133.5)
  line L64 (185.5, 126.5607) -> (185.5, 129.7925)
  line L65 (184.05, 138.5) -> (184.05, 137.0107)
  line L66 (180.5, 127) -> (181.5, 127)
  line L67 (182.9893, 124.05) -> (185.5, 126.5607)
  line L68 (180.5, 126.5) -> (180.5, 127)
  line L69 (186.5, 139.5) -> (187, 139.5)
  line L70 (181.5, 133) -> (181.5, 135.95)
  line L71 (187, 120.5) -> (187, 121.5)
  line L72 (187, 139.5) -> (187, 138.5)
  line L73 (180, 133.5) -> (180, 138.5)
  line L74 (186.5607, 134.5) -> (189.7925, 134.5)
  line L75 (193, 138.5) -> (195.95, 138.5)
  line L76 (193, 139.5) -> (193, 138.5)
  line L77 (180, 121.5) -> (180, 126.5)
  line L78 (195.95, 138.5) -> (195.95, 137.0107)
  line L79 (195.95, 121.5) -> (195.95, 122.9893)
  line L80 (193, 139.5) -> (193.5, 139.5)
  line L81 (182.9893, 135.95) -> (185.5, 133.4393)
  line L82 (193, 120.5) -> (193, 121.5)
  line L83 (184.05, 121.5) -> (184.05, 122.9893)
  line L84 (187, 138.5) -> (184.05, 138.5)
  line L85 (193, 121.5) -> (195.95, 121.5)
  line L86 (197.0107, 124.05) -> (194.5, 126.5607)
  line L87 (195.95, 122.9893) -> (193.4393, 125.5)
  line L88 (194.5, 133.4393) -> (194.5, 130.2075)
  line L89 (181.5, 127) -> (181.5, 124.05)
  line L90 (180.5, 133) -> (181.5, 133)
  line L91 (184.05, 137.0107) -> (186.5607, 134.5)
  line L92 (181.5, 135.95) -> (182.9893, 135.95)
  line L93 (186.5, 140) -> (186.5, 139.5)
  line L94 (195.95, 137.0107) -> (193.4393, 134.5)
  line L95 (193.5, 120.5) -> (193, 120.5)
  line L96 (193.5, 140) -> (193.5, 139.5)
  line L97 (184.05, 122.9893) -> (186.5607, 125.5)
  line L98 (186.5, 120) -> (181.5, 120)
  line L99 (193.5, 120) -> (193.5, 120.5)
  line L100 (186.5607, 125.5) -> (189.7925, 125.5)
  line L101 (181.5, 124.05) -> (182.9893, 124.05)
  line L102 (197.0107, 121.4935) -> (202.9893, 121.4935)
  line L103 (197.0107, 124.05) -> (197.0107, 121.4935)
  line L104 (202.9893, 124.05) -> (202.9893, 121.4935)
  line L105 (202.9893, 138.5) -> (197.0107, 138.5)
  line L106 (197.0107, 135.95) -> (197.0107, 138.5)
  line L107 (202.9893, 135.95) -> (202.9893, 138.5)
  circle A0 centre (210, 130) radius 2.74
  circle A1 centre (190, 130) radius 2.74
  arc A2 (205.5, 129.7925) -> (205.5, 130.2075) centre (205.5, 130) ccw
  arc A3 (220, 138.5) -> (218.5, 140) centre (218.5, 138.5) ccw
  arc A4 (209.7925, 134.5) -> (210.2075, 134.5) centre (210, 134.5) ccw
  arc A5 (218.5, 120) -> (220, 121.5) centre (218.5, 121.5) ccw
  arc A6 (210.2075, 125.5) -> (209.7925, 125.5) centre (210, 125.5) ccw
  arc A7 (214.5, 130.2075) -> (214.5, 129.7925) centre (214.5, 130) ccw
  arc A8 (185.5, 129.7925) -> (185.5, 130.2075) centre (185.5, 130) ccw
  arc A9 (181.5, 140) -> (180, 138.5) centre (181.5, 138.5) ccw
  arc A10 (194.5, 130.2075) -> (194.5, 129.7925) centre (194.5, 130) ccw
  arc A11 (190.2075, 125.5) -> (189.7925, 125.5) centre (190, 125.5) ccw
  arc A12 (189.7925, 134.5) -> (190.2075, 134.5) centre (190, 134.5) ccw
  arc A13 (180, 121.5) -> (181.5, 120) centre (181.5, 121.5) ccw
  point P0 (200, 130)
  dimension "d17" = 1.5
  constraint coincident L4 L48.start
  measures "d17" distance of L3 L85
extrude "Extrude7" add sketch "Sketch7" along normal blind 200 separate body makes body 7
sketch "Sketch8" plane through (0, 0, 40) normal (0, 0, 1) x (1, 0, 0)
  line L0 (5.5, 203.4393) -> (5.5, 200.2075)
  line L1 (18.5, 203) -> (18.5, 205.95)
  line L2 (6.5607, 195.5) -> (9.7925, 195.5)
  line L3 (0, 203.5) -> (0, 208.5)
  line L4 (0.5, 203) -> (0.5, 203.5)
  line L5 (15.95, 208.5) -> (15.95, 207.0107)
  line L6 (13.5, 210) -> (18.5, 210)
  line L7 (0, 196.5) -> (0.5, 196.5)
  line L8 (13.4393, 195.5) -> (10.2075, 195.5)
  line L9 (20, 196.5) -> (19.5, 196.5)
  line L10 (13.5, 190) -> (13.5, 190.5)
  line L11 (18.5, 194.05) -> (17.0107, 194.05)
  line L12 (2.9893, 194.05) -> (5.5, 196.5607)
  line L13 (0, 191.5) -> (0, 196.5)
  line L14 (19.5, 197) -> (18.5, 197)
  line L15 (4.05, 191.5) -> (4.05, 192.9893)
  line L16 (15.95, 207.0107) -> (13.4393, 204.5)
  line L17 (4.05, 208.5) -> (4.05, 207.0107)
  line L18 (1.5, 205.95) -> (2.9893, 205.95)
  line L19 (15.95, 191.5) -> (15.95, 192.9893)
  line L20 (7, 191.5) -> (4.05, 191.5)
  line L21 (19.5, 203.5) -> (19.5, 203)
  line L22 (19.5, 197) -> (19.5, 196.5)
  line L23 (18.5, 197) -> (18.5, 194.05)
  line L24 (7, 209.5) -> (7, 208.5)
  line L25 (13, 190.5) -> (13, 191.5)
  line L26 (6.5, 190) -> (1.5, 190)
  line L27 (6.5, 209.5) -> (7, 209.5)
  line L28 (20, 196.5) -> (20, 191.5)
  line L29 (14.5, 196.5607) -> (14.5, 199.7925)
  line L30 (15.95, 192.9893) -> (13.4393, 195.5)
  line L31 (18.5, 205.95) -> (17.0107, 205.95)
  line L32 (5.5, 196.5607) -> (5.5, 199.7925)
  line L33 (7, 190.5) -> (6.5, 190.5)
  line L34 (6.5, 210) -> (6.5, 209.5)
  line L35 (13, 209.5) -> (13.5, 209.5)
  line L36 (4.05, 207.0107) -> (6.5607, 204.5)
  line L37 (13, 209.5) -> (13, 208.5)
  line L38 (17.0107, 194.05) -> (14.5, 196.5607)
  line L39 (0, 203.5) -> (0.5, 203.5)
  line L40 (1.5, 210) -> (6.5, 210)
  line L41 (1.5, 197) -> (1.5, 194.05)
  line L42 (1.5, 194.05) -> (2.9893, 194.05)
  line L43 (13, 191.5) -> (15.95, 191.5)
  line L44 (0.5, 196.5) -> (0.5, 197)
  line L45 (6.5607, 204.5) -> (9.7925, 204.5)
  line L46 (13.5, 190.5) -> (13, 190.5)
  line L47 (13, 208.5) -> (15.95, 208.5)
  line L48 (2.9893, 205.95) -> (5.5, 203.4393)
  line L49 (13.5, 210) -> (13.5, 209.5)
  line L50 (20, 203.5) -> (19.5, 203.5)
  line L51 (7, 190.5) -> (7, 191.5)
  line L52 (6.5, 190) -> (6.5, 190.5)
  line L53 (1.5, 203) -> (1.5, 205.95)
  line L54 (4.05, 192.9893) -> (6.5607, 195.5)
  line L55 (19.5, 203) -> (18.5, 203)
  line L56 (0.5, 197) -> (1.5, 197)
  line L57 (20, 208.5) -> (20, 203.5)
  line L58 (17.0107, 205.95) -> (14.5, 203.4393)
  line L59 (0.5, 203) -> (1.5, 203)
  line L60 (18.5, 190) -> (13.5, 190)
  line L61 (7, 208.5) -> (4.05, 208.5)
  line L62 (13.4393, 204.5) -> (10.2075, 204.5)
  line L63 (14.5, 203.4393) -> (14.5, 200.2075)
  circle A0 centre (10, 200) radius 2.74
  arc A1 (20, 208.5) -> (18.5, 210) centre (18.5, 208.5) ccw
  arc A2 (9.7925, 204.5) -> (10.2075, 204.5) centre (10, 204.5) ccw
  arc A3 (18.5, 190) -> (20, 191.5) centre (18.5, 191.5) ccw
  arc A4 (14.5, 200.2075) -> (14.5, 199.7925) centre (14.5, 200) ccw
  arc A5 (1.5, 210) -> (0, 208.5) centre (1.5, 208.5) ccw
  arc A6 (0, 191.5) -> (1.5, 190) centre (1.5, 191.5) ccw
  arc A7 (5.5, 199.7925) -> (5.5, 200.2075) centre (5.5, 200) ccw
  arc A8 (10.2075, 195.5) -> (9.7925, 195.5) centre (10, 195.5) ccw
  line L64 (293.4393, 204.5) -> (290.2075, 204.5)
  line L65 (286.5, 190) -> (281.5, 190)
  arc A9 (300, 208.5) -> (298.5, 210) centre (298.5, 208.5) ccw
  line L66 (281.5, 194.05) -> (282.9893, 194.05)
  line L67 (293, 190.5) -> (293, 191.5)
  line L68 (293.4393, 195.5) -> (290.2075, 195.5)
  line L69 (280, 203.5) -> (280.5, 203.5)
  line L70 (280, 203.5) -> (280, 208.5)
  line L71 (295.95, 191.5) -> (295.95, 192.9893)
  line L72 (281.5, 210) -> (286.5, 210)
  line L73 (295.95, 208.5) -> (295.95, 207.0107)
  line L74 (299.5, 197) -> (298.5, 197)
  line L75 (281.5, 203) -> (281.5, 205.95)
  line L76 (280.5, 203) -> (281.5, 203)
  line L77 (293.5, 190.5) -> (293, 190.5)
  line L78 (286.5607, 195.5) -> (289.7925, 195.5)
  line L79 (299.5, 203.5) -> (299.5, 203)
  line L80 (299.5, 197) -> (299.5, 196.5)
  line L81 (300, 208.5) -> (300, 203.5)
  line L82 (287, 209.5) -> (287, 208.5)
  line L83 (286.5, 209.5) -> (287, 209.5)
  line L84 (287, 208.5) -> (284.05, 208.5)
  line L85 (300, 196.5) -> (300, 191.5)
  line L86 (286.5607, 204.5) -> (289.7925, 204.5)
  arc A10 (294.5, 200.2075) -> (294.5, 199.7925) centre (294.5, 200) ccw
  arc A11 (298.5, 190) -> (300, 191.5) centre (298.5, 191.5) ccw
  line L87 (282.9893, 194.05) -> (285.5, 196.5607)
  line L88 (297.0107, 194.05) -> (294.5, 196.5607)
  line L89 (295.95, 207.0107) -> (293.4393, 204.5)
  line L90 (285.5, 203.4393) -> (285.5, 200.2075)
  line L91 (281.5, 205.95) -> (282.9893, 205.95)
  line L92 (293, 208.5) -> (295.95, 208.5)
  line L93 (284.05, 207.0107) -> (286.5607, 204.5)
  arc A12 (290.2075, 195.5) -> (289.7925, 195.5) centre (290, 195.5) ccw
  line L94 (294.5, 203.4393) -> (294.5, 200.2075)
  line L95 (295.95, 192.9893) -> (293.4393, 195.5)
  line L96 (287, 190.5) -> (287, 191.5)
  line L97 (284.05, 192.9893) -> (286.5607, 195.5)
  line L98 (281.5, 197) -> (281.5, 194.05)
  line L99 (298.5, 197) -> (298.5, 194.05)
  line L100 (287, 191.5) -> (284.05, 191.5)
  line L101 (297.0107, 205.95) -> (294.5, 203.4393)
  line L102 (280, 191.5) -> (280, 196.5)
  arc A13 (280, 191.5) -> (281.5, 190) centre (281.5, 191.5) ccw
  line L103 (280.5, 197) -> (281.5, 197)
  line L104 (293, 209.5) -> (293.5, 209.5)
  line L105 (293.5, 210) -> (298.5, 210)
  line L106 (280.5, 196.5) -> (280.5, 197)
  line L107 (300, 196.5) -> (299.5, 196.5)
  line L108 (286.5, 190) -> (286.5, 190.5)
  line L109 (287, 190.5) -> (286.5, 190.5)
  line L110 (280, 196.5) -> (280.5, 196.5)
  line L111 (293, 209.5) -> (293, 208.5)
  line L112 (298.5, 203) -> (298.5, 205.95)
  line L113 (284.05, 191.5) -> (284.05, 192.9893)
  line L114 (294.5, 196.5607) -> (294.5, 199.7925)
  circle A14 centre (290, 200) radius 2.74
  line L115 (285.5, 196.5607) -> (285.5, 199.7925)
  line L116 (293.5, 210) -> (293.5, 209.5)
  line L117 (299.5, 203) -> (298.5, 203)
  line L118 (282.9893, 205.95) -> (285.5, 203.4393)
  line L119 (286.5, 210) -> (286.5, 209.5)
  arc A15 (289.7925, 204.5) -> (290.2075, 204.5) centre (290, 204.5) ccw
  line L120 (284.05, 208.5) -> (284.05, 207.0107)
  arc A16 (281.5, 210) -> (280, 208.5) centre (281.5, 208.5) ccw
  line L121 (293, 191.5) -> (295.95, 191.5)
  line L122 (298.5, 190) -> (293.5, 190)
  line L123 (298.5, 194.05) -> (297.0107, 194.05)
  line L124 (280.5, 203) -> (280.5, 203.5)
  line L125 (293.5, 190) -> (293.5, 190.5)
  line L126 (298.5, 205.95) -> (297.0107, 205.95)
  line L127 (300, 203.5) -> (299.5, 203.5)
  arc A17 (285.5, 199.7925) -> (285.5, 200.2075) centre (285.5, 200) ccw